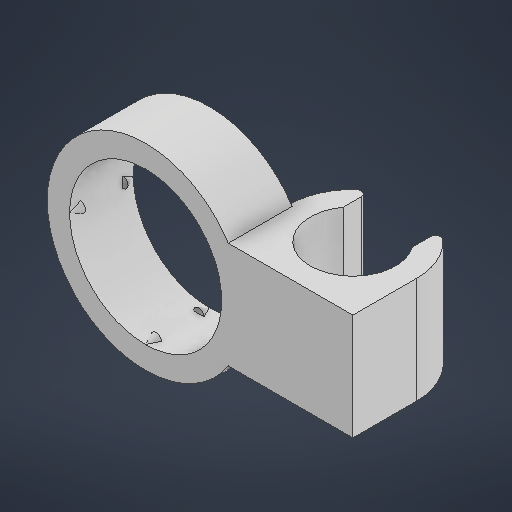
# Autodesk Inventor part: AgarreColganteCabina_v02
Saved by Autodesk Inventor 2026.1 (Build 301233020, 233B)
## iProperties
Created: 2025-11-02
Part Number: AgarreColganteCabina_v02
Material: Generic
Document SubType Name: Modeling
Designer: Tito Luyo Murata
Density: 1 g/cm^3
Appearance: Default
Author: Tito Luyo Murata
Autodesk Inventor part; units mm, degrees
ref_plane "YZ Plane" through (0, 0, 0) normal (1, 0, 0) x (0, 1, 0)
ref_plane "XZ Plane" through (0, 0, 0) normal (0, 1, 0) x (-1, 0, 0)
ref_plane "XY Plane" through (0, 0, 0) normal (0, 0, 1) x (1, 0, 0)
sketch "Sketch5" plane through (0, 0, 0) normal (0, 1, 0) x (-1, 0, 0)
  line L0 (0, 0) -> (-12, 0)
  line L1 (-12, 0) -> (-12, -12)
  line L2 (-12, -12) -> (0, -12)
  line L3 (0, -12) -> (0, 0)
  circle A0 centre (-6, -6) radius 4
  circle A1 centre (-6, -6) radius 6
  line L4 (-6, -6) -> (-6, -14) construction
  line L5 (-2.75, -8) -> (-9.25, -8)
  line L6 (-9.25, -8) -> (-9.25, -12)
  line L7 (-9.25, -12) -> (-2.75, -12)
  line L8 (-2.75, -12) -> (-2.75, -8)
  line L9 (-2.75, -8) -> (-9.25, -12) construction
  line L10 (-9.25, -8) -> (-2.75, -12) construction
  point P0 (-6, -10)
  point P1 (-12, -6)
  point P2 (-9.25, -11.0436)
  point P3 (-9.25, -8.3318)
  point P4 (-2.75, -8.3318)
  point P5 (-2.75, -11.0436)
  point P6 (0, -6)
  dimension "d10" = 12
  dimension "d11" = 12
  dimension "d12" = 8
  dimension "d13" = 12
  dimension "d14" = 8
  dimension "d15" = 6.5
  constraints: 22 end point, 4 parallel, 3 midpoint, 2 centre point, 2 horizontal, 2 perpendicular, 1 coincident, 1 point on line, 1 vertical
  measures "d10" distance of L2.end L1.end
  measures "d11" distance of L1.end L0.end
  measures "d12" diameter of A0
  measures "d13" diameter of A1
  measures "d14" distance of L4.start L4.end
  measures "d15" distance of L7.end L6.end
extrude "Extrusion3" add sketch "Sketch5" along normal blind 10 contours L3 A1 L0 | A1 L1 L0 | A1 L8 A0 L6 picked at (-9.6317, -9.82)
fillet "Fillet1" radius 0.5 2 edges at (2.75, 5, -11.0436) (9.25, 5, -11.0436)
sketch "Sketch6" plane through (0, 0, 0) normal (0, 0, 1) x (1, 0, 0)
  circle A0 centre (-7.5, 5) radius 9.25
  line L0 (0, 5) -> (0, 10)
  circle A1 centre (-7.5, 5) radius 7.15
  line L1 (12, 0) -> (12, 10) construction
  line L2 (12, 5) -> (-28, 5) construction
  line L3 (12, 5) -> (52, 5) construction
  dimension "d19" = 18.5
  dimension "d22" = 14.3
  dimension "d35" = 7.5
  dimension "d43" = 40
  dimension "d44" = 180
  constraints: 6 end point, 2 centre point, 1 coincident, 1 collinear, 1 horizontal, 1 midpoint, 1 perpendicular, 1 point on line
  measures "d19" diameter of A0
  measures "d22" diameter of A1
  measures "d35" distance from line of A0.centre L0
  measures "d43" distance of L2.start L2.end
  measures "d44" angle of L2 L3
extrude "Extrusion4" add sketch "Sketch6" against normal blind 6
ref_plane "Work Plane3" through (0, 5, 0) normal (0, 1, 0) x (1, 0, 0)
sketch "Sketch9" plane through (0, 5, 0) normal (0, 1, 0) x (1, 0, 0)
  line L0 (-14.65, 6) -> (-0.35, 6) projected
  line L1 (-0.35, 6) -> (-0.35, 5)
  line L2 (-0.35, 6) -> (-0.35, 0) projected
  line L3 (-0.35, 6) -> (0.65, 6) construction
  line L4 (-0.35, 5) -> (-0.85, 5)
  line L5 (-0.85, 5) -> (-0.35, 6)
  point P0 (0, 0)
  dimension "d36" = 1
  dimension "d37" = 90
  dimension "d38" = 0.5
  constraints: 8 end point, 2 perpendicular, 1 collinear, 1 horizontal
  measures "d36" distance of L0.end L1.end
  measures "d37" angle of L1 L3
  measures "d38" distance of L1.end L4.end
revolve "Revolution2" add sketch "Sketch9" angle 360 about axis through (-0.35, 5, -6) along (0, 0, 1)
pattern_circular "Circular Pattern2" count 4 over 360 about axis through (-7.5, 5, 0) along (0, 0, -1) of "Revolution2"
ref_plane "Work Plane4" through (0, 0, -3) normal (0, 0, -1) x (-1, 0, 0)
mirror "Mirror2" about plane through (0, 0, -3) normal (0, 0, -1) of "Revolution2", "Circular Pattern2"
equation "\"tol\" = 0.3"
equation "\"tol_int\" = 0.1"
body "Solid2"
